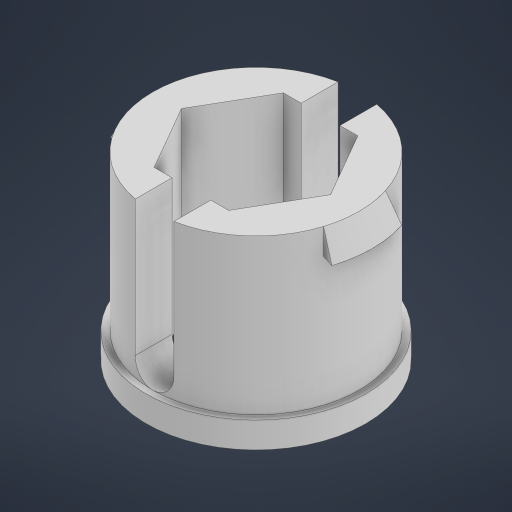
# Autodesk Inventor part: 5mmHexInsert
Saved by Autodesk Inventor 2023 (Build 270158000, 158)
## iProperties
Created: 2023-02-25
Part Number: 5mmHexInsert
Material: Generic
Document SubType Name: Modeling
Designer: izack
Density: 1 g/cm^3
Appearance: Default
Author: izack
Autodesk Inventor part; units mm, degrees
ref_plane "YZ Plane" through (0, 0, 0) normal (1, 0, 0) x (0, 1, 0)
ref_plane "XZ Plane" through (0, 0, 0) normal (0, 1, 0) x (-1, 0, 0)
sketch "Sketch1" plane through (0, 0, 0) normal (0, 1, 0) x (-1, 0, 0)
  circle A0 centre (0, 0) radius 4
  circle A1 centre (0, 0) radius 2.5 construction
  line L0 (1.4434, 2.5) -> (2.8868, 0)
  line L1 (2.8868, 0) -> (1.4434, -2.5)
  line L2 (1.4434, -2.5) -> (-1.4434, -2.5)
  line L3 (-1.4434, -2.5) -> (-2.8868, 0)
  line L4 (-2.8868, 0) -> (-1.4434, 2.5)
  line L5 (-1.4434, 2.5) -> (1.4434, 2.5)
  line L6 (0, -2.5) -> (0, -4) construction
  line L7 (0.75, -2.5) -> (0.75, -3.9291)
  line L8 (-0.75, -2.5) -> (-0.75, -3.9291)
  line L9 (2.8868, 0) -> (-2.8868, 0) construction
  line L10 (0.75, 2.5) -> (0.75, 3.9291)
  line L11 (-0.75, 2.5) -> (-0.75, 3.9291)
  point P0 (0, 2.5)
  point P1 (-0.75, 2.5)
  point P2 (-0.75, 3.9291)
  point P3 (0.75, 3.9291)
  point P4 (0.75, 2.5)
  dimension "d1" = 5
  dimension "d0" = 8
  dimension "d2" = 0.75
  dimension "d3" = 0.75
  constraints: 24 end point, 4 symmetric about line, 3 coincident, 3 point on circle, 2 horizontal, 2 midpoint, 2 point on line, 1 centre point, 1 parallel, 1 perpendicular, 1 vertical, 1 vertical alignment, 15 other
  measures "d0" diameter of A0
  measures "d2" distance between parallel lines of L6 L8
  measures "d3" distance between parallel lines of L6 L7
extrude "Extrusion1" add sketch "Sketch1" along normal blind 6 contours A0 L7 L2 L1 L0 L5 L10 | L11 L5 L4 L3 L2 L8 A0
sketch "Sketch2" plane through (0, 0, 0) normal (0, -1, 0) x (1, 0, 0)
  circle A0 centre (0, 0) radius 4.25
  line L0 (2.8868, 0) -> (1.4434, 2.5) projected
  line L1 (2.8868, 0) -> (1.4434, -2.5)
  line L2 (1.4434, -2.5) -> (-1.4434, -2.5)
  line L3 (-1.4434, -2.5) -> (-2.8868, 0)
  line L4 (-2.8868, 0) -> (-1.4434, 2.5)
  line L5 (-1.4434, 2.5) -> (1.4434, 2.5)
  line L6 (1.4434, 2.5) -> (2.8868, 0)
  dimension "d6" = 8.5
  constraints: 12 end point, 2 coincident, 1 centre point, 13 other
  measures "d6" diameter of A0
extrude "Extrusion2" add sketch "Sketch2" along normal blind 1
ref_plane "Work Plane1" through (0.75, 6, 0) normal (0, 0, 1) x (1, 0, 0)
sketch "Sketch3" plane through (0.75, 6, 0) normal (0, 0, 1) x (1, 0, 0)
  line L0 (3.25, 0) -> (0, 0) projected
  line L1 (3.25, 0) -> (3.25, -1)
  line L2 (3.25, -6) -> (3.25, 0) projected
  line L3 (3.25, -1) -> (3.75, -1)
  line L4 (3.75, -1) -> (3.25, 0)
  line L5 (3.25, 0) -> (2.9426, 0)
  line L6 (2.9426, 0) -> (2.9426, -1)
  line L7 (2.9426, -1) -> (3.25, -1)
  line L8 (-0.75, -6) -> (-0.75, 0) construction
  line L9 (-4.75, 0) -> (-1.5, 0)
  line L10 (-4.75, 0) -> (-4.75, -1)
  line L11 (-4.75, -1) -> (-5.25, -1)
  line L12 (-5.25, -1) -> (-4.75, 0)
  line L13 (-4.4426, 0) -> (-4.4426, -1)
  line L14 (-4.4426, -1) -> (-4.75, -1)
  dimension "d9" = 1
  dimension "d10" = 0.5
  constraints: 26 end point, 7 symmetric about line, 5 point on line, 2 perpendicular, 1 parallel, 1 vertical
  measures "d9" distance of L0.start L1.end
  measures "d10" distance of L1.end L3.end
revolve "Revolution1" add sketch "Sketch3" angle 35 mid plane about axis through (0, 0, 0) along (0, 1, 0) contours L4 L3 L1 | L10 L11 L12
fillet "Fillet1" radius 0.75 4 edges at (0.75, 0, 3.2145) (-0.75, 0, 3.2145) (0.75, 0, -3.2145) (-0.75, 0, -3.2145)
body "Solid1"
